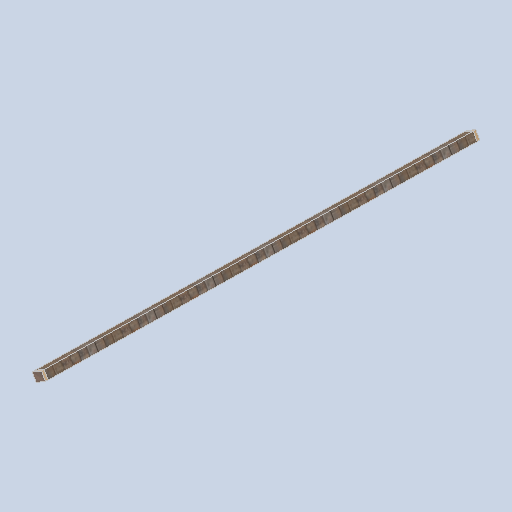
# Autodesk Inventor part: support_beam_segment_0105
Saved by Autodesk Inventor 2024.2 (Build 282272000, 272)
## iProperties
Created: 2024-05-20
Part Number: support_beam_segment_0105
Material: Wood (Maple)
Document SubType Name: Modeling
Designer: LOSTER_1
Density: 0.67 g/cm^3
Appearance: Natural Maple - Glossy Dark Tint
Author: LOSTER_1
Autodesk Inventor part; units mm, degrees
ref_plane "YZ Plane" through (0, 0, 0) normal (1, 0, 0) x (0, 1, 0)
ref_plane "XZ Plane" through (0, 0, 0) normal (0, 1, 0) x (-1, 0, 0)
sketch "Sketch1" plane through (0, 0, 0) normal (0, 0, 1) x (1, 0, 0)
  line L0 (-43.6494, -53.1082) -> (-216.8545, -153.1082)
  line L1 (-216.8657, -153.1146) -> (-141.8657, -283.0184)
  line L2 (31.3394, -183.0184) -> (-43.6606, -53.1146)
  line L3 (-141.8545, -283.012) -> (31.3506, -183.012)
  line L4 (-141.8433, -283.0055) -> (31.3394, -183.0184)
  line L5 (31.3394, -183.0184) -> (-43.6606, -53.1146)
  line L6 (-43.6606, -53.1146) -> (-216.8433, -153.1017)
  line L7 (-216.8433, -153.1017) -> (-141.8433, -283.0055)
  line L8 (-141.8433, -283.0055) -> (-43.6606, -53.1146) construction
  line L9 (31.3394, -183.0184) -> (-216.8433, -153.1017) construction
  point P0 (-92.7519, -168.0601)
  constraints: 20 end point, 2 midpoint, 2 parallel, 1 perpendicular
ref_plane "Work Plane2" through (0, 0, 8101) normal (0, 0, 1) x (1, 0, 0)
ref_plane "Work Plane1" through (0, 0, 0) normal (0, 0, 1) x (1, 0, 0)
sketch "Sketch2" plane through (0, 0, 8101) normal (0, 0, 1) x (1, 0, 0)
  line L0 (137.5706, 278.3594) -> (-35.6372, 178.364) projected
  line L1 (212.5671, 148.4536) -> (137.5706, 278.3594) projected
  line L2 (39.3594, 48.4582) -> (212.5671, 148.4536) projected
  line L3 (-35.6372, 178.364) -> (39.3594, 48.4582) projected
  line L4 (212.5671, 148.4536) -> (39.3594, 48.4582)
  line L5 (39.3594, 48.4582) -> (-35.6372, 178.364)
  line L6 (-35.6372, 178.364) -> (137.5706, 278.3594)
  line L7 (137.5706, 278.3594) -> (212.5671, 148.4536)
  line L8 (212.5671, 148.4536) -> (-35.6372, 178.364) construction
  line L9 (39.3594, 48.4582) -> (137.5706, 278.3594) construction
  point P0 (0, 0)
  point P1 (88.465, 163.4088)
  constraints: 12 end point, 2 midpoint, 2 parallel, 1 perpendicular
loft "Loft1" add profiles "Sketch2", "Sketch1"
sketch "Sketch3" plane through (-43.6606, -53.1146, 0) normal (0, 0, -1) x (-0.866, -0.5, 0)
  line L0 (0, 0) -> (199.9742, 0) projected
  line L1 (0, -150) -> (0, 0) projected
  line L2 (199.9742, -150) -> (0, -150) projected
  line L3 (199.9742, 0) -> (199.9742, -150) projected
  point P0 (-64.3685, 24.1683)
sketch "Sketch4" plane through (-35.6372, 178.364, 8101) normal (0, 0, 1) x (0.866, 0.5, 0)
  line L0 (200, 0) -> (0, 0) projected
  line L1 (0, 0) -> (0, -150) projected
  line L2 (0, -150) -> (200, -150) projected
  line L3 (200, -150) -> (200, 0) projected
  point P0 (-58.3147, -172.2879)
extrude "Extrusion1" add sketch "Sketch3" along normal blind 50
extrude "Extrusion2" add sketch "Sketch4" along normal blind 50
body "Solid1"
